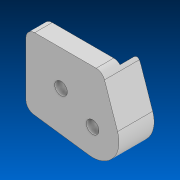
# Autodesk Inventor part: Elevator Tensioner
Saved by Autodesk Inventor 2022 (Build 260153000, 153)
## iProperties
Created: 2022-04-08
Part Number: Elevator Tensioner
Material: Generic
Document SubType Name: Modeling
Designer: score_nygvs6w
Density: 1 g/cm^3
Appearance: Default
Author: score_nygvs6w
Autodesk Inventor part; units mm, degrees
ref_plane "YZ Plane" through (0, 0, 0) normal (1, 0, 0) x (0, 1, 0)
ref_plane "XZ Plane" through (0, 0, 0) normal (0, 1, 0) x (-1, 0, 0)
ref_plane "XY Plane" through (0, 0, 0) normal (0, 0, 1) x (1, 0, 0)
sketch "Sketch1" plane through (0, 0, 0) normal (0, 0, 1) x (1, 0, 0)
  line L0 (12.7, -12.7) -> (-12.7, -12.7)
  line L1 (-12.7, -12.7) -> (-12.7, 12.7)
  line L2 (-12.7, 12.7) -> (12.7, 12.7)
  line L3 (12.7, 12.7) -> (12.7, -12.7)
  line L4 (12.7, -12.7) -> (-12.7, 12.7) construction
  line L5 (-12.7, -12.7) -> (12.7, 12.7) construction
  circle A0 centre (11.43, -6.35) radius 9.525
  line L6 (12.7, 12.7) -> (14.986, 12.7)
  line L7 (14.986, 12.7) -> (14.986, -15.1863)
  line L8 (14.986, -12.7) -> (12.7, -12.7)
  line L9 (12.7, -12.7) -> (12.7, 12.7) construction
  line L10 (6.6364, -7.4249) -> (8.1023, -2.736) construction
  line L11 (8.1023, -2.736) -> (12.8959, -1.6611) construction
  line L12 (12.8959, -1.6611) -> (16.2236, -5.2751) construction
  line L13 (16.2236, -5.2751) -> (14.7577, -9.964) construction
  line L14 (14.7577, -9.964) -> (9.9641, -11.0389) construction
  line L15 (9.9641, -11.0389) -> (6.6364, -7.4249) construction
  circle A1 centre (11.43, -6.35) radius 2.286
  circle A2 centre (11.43, -6.35) radius 4.0005
  circle A3 centre (0, 0) radius 2.286
  line L16 (10.1541, -15.7892) -> (-12.7, -12.7)
  line L17 (14.986, 12.7) -> (20.4433, -3.27)
  point P0 (14.986, -9.2337)
  point P1 (14.986, -4.5173)
  point P2 (14.986, -8.1827)
  point P3 (12.1553, 12.7)
  point P4 (-5.8053, 12.7)
  point P5 (4.3305, -12.7)
  point P6 (12.7, 3.09)
  point P7 (14.986, 2.4863)
  dimension "d0" = 25.4
  dimension "d1" = 25.4
  dimension "d3" = 19.05
  dimension "d5" = 8.509
  dimension "d6" = 4.572
  dimension "d13" = 8.001
  dimension "d17" = 4.572
  dimension "d19" = 2.286
  dimension "d26" = 6.35
  dimension "d27" = 11.43
  constraints: 36 end point, 4 centre point, 4 coincident, 4 parallel, 3 midpoint, 3 point on circle, 2 horizontal, 2 perpendicular, 2 tangent, 1 collinear, 1 point on line, 13 other
  measures "d0" distance between parallel lines of L3 L1
  measures "d1" distance between parallel lines of L0 L2
  measures "d3" diameter of A0
  measures "d5" distance between parallel lines of L11 L14
  measures "d6" diameter of A1
  measures "d13" diameter of A2
  measures "d17" diameter of A3
  measures "d19" distance between parallel lines of L3 L7
  measures "d26" vertical distance of A0.centre point (0, 0)
  measures "d27" horizontal distance of point (11.43, -6.35) point (0, 0)
extrude "Extrusion1" add sketch "Sketch1" along normal blind 6.35 contours L8 L7 A0 L0 | L0 A0 L3 A2 | L3 A2 L7 L8 | A0 L16 L0 | L0 L1 L2 L3 A0 | A2 L3 A1 | L3 A1 A2 L7 | L7 A2 A0 | A0 L7 A2 L3 | L3 L6 L7 A0 | L7 A2 | L7 L17 A0
extrude "Extrusion2" add sketch "Sketch1" against normal blind 6.35 contours L7 A2 A0 | L7 L17 A0
extrude "Extrusion3" cut sketch "Sketch1" along normal blind 2.54 contours A2 L3 A1 | L3 A1 A2 L7 | L7 A2
fillet "Fillet2" radius 3.175 3 edges at (14.986, 12.7, 3.175) (-12.7, -12.7, 3.175) (-12.7, 12.7, 3.175)
fillet "Fillet1" radius 1.27 1 edges at (14.986, 3.6136, -6.35)
body "Solid1"
